Autodesk Fusion 360 part; units mm, degrees
(part 2 of 2)
  constraint parallel L118 L151
  constraint coincident P35 L167
  constraint coincident P35 L166
  constraint coincident P35 A26.centre
  constraint horizontal L165
  constraint perpendicular L135 L165
  constraint parallel L165 L187
  constraint parallel L128 L135
  constraint coincident P47 L131
  constraint coincident P47 L144
  constraint coincident P47 A24.centre
  constraint horizontal L111
  constraint perpendicular L108 L111
  constraint parallel L111 L113
  constraint parallel L108 L110
  constraint coincident P52 L114
  constraint coincident P52 L112
  constraint coincident P52 A18.centre
  constraint horizontal L115
  constraint perpendicular L115 L122
  constraint parallel L115 L117
  constraint parallel L121 L122
  constraint coincident P50 L119
  constraint coincident P50 L120
  constraint coincident P50 A19.centre
  constraint horizontal L116
  constraint perpendicular L116 L137
  constraint parallel L116 L180
  constraint parallel L136 L137
  constraint coincident P28 L134
  constraint coincident P28 L130
  constraint coincident P28 A21.centre
  constraint horizontal L161
  constraint perpendicular L161 L181
  constraint parallel L161 L164
  constraint parallel L181 L206
  constraint coincident P40 L154
  constraint coincident P40 L155
  constraint coincident P40 A29.centre
  constraint horizontal L195
  constraint perpendicular L195 L204
  constraint parallel L190 L195
  constraint parallel L194 L204
  constraint coincident P46 L197
  constraint coincident P46 L201
  constraint coincident P46 A34.centre
  constraint horizontal L193
  constraint perpendicular L186 L193
  constraint parallel L172 L193
  constraint parallel L175 L186
  constraint coincident P53 L189
  constraint coincident P53 L192
  constraint coincident P53 A33.centre
  constraint horizontal L216
  constraint perpendicular L216 L217
  constraint parallel L216 L218
  constraint parallel L217 L219
  constraint coincident L220 P56
  constraint coincident L221 P56
  constraint coincident P56 A36.centre
  measures "d3" distance of L1.end L2.end
  measures "d4" distance of L0.end L1.end
  measures "d5" diameter of A0
  measures "d6" distance of L6.end L7.end
  measures "d7" distance of L6.end L6.start
  measures "d8" diameter of A1
  measures "d9" distance of L14.end L12.end
  measures "d10" distance of L12.start L14.end
  measures "d11" diameter of A2
  measures "d12" distance of L31.start L28.end
  measures "d13" distance of L31.start L28.start
  measures "d14" diameter of A5
  measures "d15" distance of L24.end L20.start
  measures "d16" distance of L26.start L24.end
  measures "d17" diameter of A4
  measures "d18" distance of L18.start L18.end
  measures "d19" distance of L18.start L19.start
  measures "d20" diameter of A3
  measures "d21" distance of L50.end L65.start
  measures "d22" distance of L50.end L50.start
  measures "d23" diameter of A10
  measures "d24" distance of L57.end L59.end
  measures "d25" distance of L59.start L57.end
  measures "d26" diameter of A8
  measures "d27" distance of L37.end L38.end
  measures "d28" distance of L37.end L38.start
  measures "d29" diameter of A6
  measures "d30" distance of L46.start L46.end
  measures "d31" distance of L47.start L46.start
  measures "d32" diameter of A7
  measures "d33" distance of L45.start L45.end
  measures "d34" distance of L45.start L51.end
  measures "d35" diameter of A9
  measures "d36" distance of L36.end L42.end
  measures "d37" distance of L36.end L41.start
  measures "d38" diameter of A11
  measures "d39" distance of L76.start L74.end
  measures "d40" distance of L74.end L77.start
  measures "d41" diameter of A13
  measures "d42" distance of L73.start L73.end
  measures "d43" distance of L73.start L72.end
  measures "d44" diameter of A12
  measures "d45" distance of L78.start L84.end
  measures "d46" distance of L79.start L84.end
  measures "d47" diameter of A14
  measures "d48" distance of L91.end L97.end
  measures "d49" distance of L91.end L96.end
  measures "d50" diameter of A15
  measures "d51" distance of L98.end L98.start
  measures "d52" distance of L101.start L98.start
  measures "d53" diameter of A17
  measures "d54" distance of L94.end L92.end
  measures "d55" distance of L94.end L90.end
  measures "d56" diameter of A16
  measures "d57" distance of L183.end L185.end
  measures "d58" distance of L183.end L185.start
  measures "d59" diameter of A32
  measures "d60" distance of L200.end L203.end
  measures "d61" distance of L199.end L200.end
  measures "d62" diameter of A35
  measures "d63" distance of L139.end L132.end
  measures "d64" distance of L139.end L132.start
  measures "d65" diameter of A23
  measures "d66" distance of L170.start L170.end
  measures "d67" distance of L171.end L170.start
  measures "d68" diameter of A31
  measures "d69" distance of L205.start L205.end
  measures "d70" distance of L205.start L173.end
  measures "d71" diameter of A30
  measures "d72" distance of L125.end L140.start
  measures "d73" distance of L125.end L138.start
  measures "d74" diameter of A22
  measures "d75" distance of L124.start L147.start
  measures "d76" distance of L152.end L147.start
  measures "d77" diameter of A27
  measures "d78" distance of L145.end L145.start
  measures "d79" distance of L145.start L146.end
  measures "d80" diameter of A28
  measures "d81" distance of L126.end L127.start
  measures "d82" distance of L126.end L126.start
  measures "d83" diameter of A25
  measures "d84" distance of L109.start L123.end
  measures "d85" distance of L123.end L123.start
  measures "d86" diameter of A20
  measures "d87" distance of L151.end L118.start
  measures "d88" distance of L151.end L151.start
  measures "d89" diameter of A26
  measures "d90" distance of L128.start L131.end
  measures "d91" distance of L135.start L131.end
  measures "d92" diameter of A24
  measures "d93" distance of L108.end L110.start
  measures "d94" distance of L108.start L108.end
  measures "d95" diameter of A18
  measures "d96" distance of L117.start L117.end
  measures "d97" distance of L117.start L115.end
  measures "d98" diameter of A19
  measures "d99" distance of L134.end L130.end
  measures "d100" distance of L134.end L116.end
  measures "d101" diameter of A21
  measures "d102" distance of L155.end L154.end
  measures "d103" distance of L155.start L154.end
  measures "d104" diameter of A29
  measures "d105" distance of L190.end L190.start
  measures "d106" distance of L195.end L190.start
  measures "d107" diameter of A34
  measures "d108" distance of L172.end L172.start
  measures "d109" distance of L186.start L172.start
  measures "d110" diameter of A33
  measures "d111" distance of L217.end L218.end
  measures "d112" distance of L216.end L217.end
  measures "d113" diameter of A36
extrude "Extrude3" add sketch "basePCB" against normal blind 10.5 contours A0 makes body 1
extrude "Extrude4" add sketch "keys" along normal blind 3.8 contours L0 L1 L2 L3 | A0 | L6 L8 L9 L10 | A1 | L13 L15 L16 L17 | A2 | L18 L22 L23 L33 | A3 | L20 L25 L27 L30 | L29 L31 L32 L34 | A4 | A5 | A6 | L39 L40 L52 L54 | L41 L43 L44 L49 | L45 L51 L62 L63 | L46 L48 L53 L55 | A7 | A8 | L50 L65 L66 L70 | A9 | A10 | L60 L61 L64 L67 | A11 | L72 L73 L75 L87 | L76 L77 L80 L88 | A12 | A13 | L78 L82 L85 L86 | A14 | L90 L93 L95 L99 | A15 | A16 | L96 L97 L104 L107 | L98 L101 L102 L105 | A17 | L108 L110 L111 L113 | L109 L123 L160 L168 | A18 | L115 L117 L121 L122 | L116 L136 L137 L180 | L118 L151 L157 L163 | A19 | L124 L147 L152 L177 | A20 | L126 L127 L158 L159 | L128 L135 L165 L187 | A21 | A22 | L133 L141 L178 L202 | L138 L140 L176 L207 | A23 | A24 | A25 | A26 | L145 L146 L150 L212 | A27 | A28 | L161 L164 L181 L206 | A29 | L170 L171 L174 L179 | L172 L175 L186 L193 | L173 L205 L210 L214 | A30 | A31 | L188 L191 L196 L198 | L190 L194 L195 L204 | A32 | A33 | L199 L203 L209 L213 | A34 | A35 | L216 L217 L218 L219 | A36 bodies 1 makes body 2 at (-44.6574, 0, -22.3613) makes body 3 at (-36.7574, 0, -22.3613) makes body 4 at (-44.6574, 0, -9.9613) makes body 5 at (29.0426, 0, 5.6053) makes body 6 at (-10.6074, 0, -19.1947) makes body 7 at (29.0426, 0, -19.1947) makes body 8 at (21.1426, 0, 5.6053) makes body 9 at (10.7426, 0, -22.3613) makes body 10 at (18.6426, 0, 17.9053) makes body 11 at (13.2426, 0, -6.7947) makes body 12 at (13.2426, 0, 5.6053) makes body 13 at (-10.6074, 0, 17.9053) makes body 14 at (44.7926, 0, 5.6053) makes body 15 at (-10.6074, 0, -6.7947) makes body 16 at (-26.3574, 0, -6.7947) makes body 17 at (1.6397, 0, 27.6219) makes body 18 at (-34.2574, 0, -6.7947) makes body 19 at (-18.4574, 0, 17.9053) makes body 20 at (-18.4574, 0, 5.6053) makes body 21 at (-26.3574, 0, 5.6053) makes body 22 at (-42.1574, 0, 5.6053) makes body 23 at (44.7926, 0, -6.7947) makes body 24 at (-10.6074, 0, 5.6053) makes body 25 at (36.9426, 0, -19.1947) makes body 26 at (13.2426, 0, 17.9053) makes body 27 at (26.4926, 0, 17.9053) makes body 28 at (29.0426, 0, -6.7947) makes body 29 at (21.1426, 0, -6.7947) makes body 30 at (36.9426, 0, -6.7947) makes body 31 at (36.9426, 0, 5.6053) makes body 32 at (21.1426, 0, -19.1947) makes body 33 at (-28.8574, 0, -22.3613) makes body 34 at (-26.3574, 0, 17.9053) makes body 35 at (44.7926, 0, -19.1947) makes body 36 at (-34.2574, 0, 5.6053) makes body 37 at (-18.4574, 0, -19.1947) makes body 38 at (-18.4574, 0, -6.7947)
extrude "Extrude5" add sketch "keys" along normal blind 7.25 contours A0 | A1 | A2 | A3 | A4 | A5 | A6 | A7 | A8 | A9 | A10 | A11 | A12 | A13 | A14 | A15 | A16 | A17 | A18 | A19 | A20 | A21 | A22 | A23 | A24 | A25 | A26 | A27 | A28 | A29 | A30 | A31 | A32 | A33 | A34 | A35 | A36 bodies 2 3 4 5 6 7 8 9 10 11 12 13 14 15 16 17 18 19 20 21 22 23 24 25 26 27 28 29 30 31 32 33 34 35 36 37 38 1
sketch "base_v2pcb" plane through (0, 0, 0) normal (0, 1, 0) x (1, 0, 0)
  line L0 (39.648, 25.534) -> (39.898, 25.534)
  line L1 (39.898, 25.534) -> (46.898, 25.534)
  line L2 (47.148, 25.284) -> (47.148, 25.534)
  line L3 (39.648, 16.284) -> (39.648, 25.284)
  line L4 (47.148, 16.034) -> (47.148, 16.284)
  line L5 (46.898, 16.034) -> (39.898, 16.034)
  line L6 (47.148, 25.284) -> (47.148, 16.284)
  line L7 (39.898, 16.034) -> (39.648, 16.034)
  line L8 (39.648, 25.284) -> (39.648, 25.534)
  line L9 (39.648, 16.034) -> (39.648, 16.284)
  line L10 (47.148, 25.534) -> (46.898, 25.534)
  line L11 (31.774, -8.754) -> (31.774, -8.504)
  line L12 (32.024, -8.754) -> (31.774, -8.754)
  line L13 (31.774, 0.746) -> (32.024, 0.746)
  line L14 (39.274, -8.754) -> (39.274, -8.504)
  line L15 (46.898, 16.034) -> (47.148, 16.034)
  line L16 (39.274, 0.496) -> (39.274, -8.504)
  line L17 (31.774, -8.504) -> (31.774, 0.496)
  line L18 (32.024, 0.746) -> (39.024, 0.746)
  line L19 (31.774, 0.496) -> (31.774, 0.746)
  line L20 (-8.224, 16.034) -> (-8.224, 16.284)
  line L21 (-8.224, 0.746) -> (-8.474, 0.746)
  line L22 (-15.474, 0.746) -> (-8.474, 0.746)
  circle A0 centre (48.514, 33.79) radius 2.45
  circle A1 centre (-48.768, 33.79) radius 2.45
  line L23 (22.472, 35.136) -> (22.472, 31.936)
  line L24 (19.846, 28.48) -> (19.846, 31.48)
  circle A2 centre (-33.782, -33.52) radius 2.45
  circle A3 centre (-42.164, 31.492) radius 2.25
  line L25 (44.066, 33.002) -> (44.066, 36.102)
  line L26 (-23.402, 31.226) -> (-23.402, 28.226)
  line L27 (32.392, 35.136) -> (22.472, 35.136)
  line L28 (-11.142, 28.226) -> (-11.142, 31.226)
  line L29 (19.846, 32.036) -> (19.846, 35.036)
  line L30 (34.764, 28.226) -> (47.024, 28.226)
  line L31 (22.472, 31.936) -> (32.392, 31.936)
  line L32 (34.764, 31.226) -> (34.764, 28.226)
  line L33 (19.846, 35.036) -> (7.586, 35.036)
  line L34 (7.586, 32.036) -> (19.846, 32.036)
  line L35 (22.472, 28.38) -> (32.392, 28.38)
  line L36 (37.966, 36.102) -> (37.966, 33.002)
  line L37 (-11.142, 31.226) -> (-23.402, 31.226)
  line L38 (47.024, 28.226) -> (47.024, 31.226)
  line L39 (7.586, 35.036) -> (7.586, 32.036)
  line L40 (32.392, 31.58) -> (22.472, 31.58)
  line L41 (37.966, 33.002) -> (44.066, 33.002)
  line L42 (7.586, 31.48) -> (7.586, 28.48)
  line L43 (44.066, 36.102) -> (37.966, 36.102)
  line L44 (32.392, 31.936) -> (32.392, 35.136)
  circle A4 centre (33.782, -33.52) radius 2.45
  line L45 (32.392, 28.38) -> (32.392, 31.58)
  line L46 (7.586, 28.48) -> (19.846, 28.48)
  line L47 (47.024, 31.226) -> (34.764, 31.226)
  line L48 (19.846, 31.48) -> (7.586, 31.48)
  line L49 (22.472, 31.58) -> (22.472, 28.38)
  line L50 (-31.172, 35.268) -> (-31.172, 28.168)
  line L51 (-37.395, 28.295) -> (-34.995, 28.295)
  line L52 (-23.402, 28.226) -> (-11.142, 28.226)
  line L53 (-34.995, 28.295) -> (-34.995, 35.395)
  line L54 (-37.395, 35.395) -> (-37.395, 28.295)
  line L55 (-31.172, 28.168) -> (-28.772, 28.168)
  line L56 (-28.772, 35.268) -> (-31.172, 35.268)
  line L57 (-28.772, 28.168) -> (-28.772, 35.268)
  line L58 (-39.97, 3.588) -> (-46.97, 3.588)
  line L59 (-39.72, 3.588) -> (-39.72, 3.838)
  line L60 (-46.97, 13.088) -> (-39.97, 13.088)
  line L61 (-39.72, 12.838) -> (-39.72, 13.088)
  line L62 (-15.658, 35.34) -> (-15.658, 32.24)
  line L63 (-12.058, 32.24) -> (-12.058, 35.34)
  line L64 (-22.77, 32.24) -> (-19.17, 32.24)
  line L65 (-34.995, 35.395) -> (-37.395, 35.395)
  line L66 (-46.97, 3.588) -> (-47.22, 3.588)
  line L67 (-22.77, 35.34) -> (-22.77, 32.24)
  line L68 (-19.17, 35.34) -> (-22.77, 35.34)
  line L69 (-47.22, 13.088) -> (-46.97, 13.088)
  line L70 (-39.97, 3.588) -> (-39.72, 3.588)
  line L71 (-15.658, 32.24) -> (-12.058, 32.24)
  line L72 (-47.22, 3.838) -> (-47.22, 12.838)
  line L73 (-39.72, 13.088) -> (-39.97, 13.088)
  line L74 (-19.17, 32.24) -> (-19.17, 35.34)
  line L75 (-47.22, 3.588) -> (-47.22, 3.838)
  line L76 (-12.058, 35.34) -> (-15.658, 35.34)
  line L77 (-39.72, 12.838) -> (-39.72, 3.838)
  line L78 (39.274, 25.284) -> (39.274, 25.534)
  line L79 (31.774, 16.034) -> (31.774, 16.284)
  line L80 (32.024, 25.534) -> (39.024, 25.534)
  line L81 (31.774, 25.284) -> (31.774, 25.534)
  line L82 (39.024, 16.034) -> (39.274, 16.034)
  line L83 (32.024, 16.034) -> (31.774, 16.034)
  line L84 (31.774, 16.284) -> (31.774, 25.284)
  line L85 (31.774, 25.534) -> (32.024, 25.534)
  line L86 (31.4, 0.746) -> (31.15, 0.746)
  line L87 (39.274, 25.534) -> (39.024, 25.534)
  line L88 (24.15, -21.05) -> (23.9, -21.05)
  line L89 (23.9, -8.754) -> (23.9, -8.504)
  line L90 (31.4, -11.8) -> (31.4, -11.55)
  line L91 (31.4, -11.55) -> (31.15, -11.55)
  line L92 (24.15, -11.55) -> (31.15, -11.55)
  line L93 (39.274, 16.034) -> (39.274, 16.284)
  line L94 (23.9, -11.8) -> (23.9, -11.55)
  line L95 (23.9, 0.746) -> (24.15, 0.746)
  line L96 (23.9, -8.504) -> (23.9, 0.496)
  line L97 (23.9, -20.8) -> (23.9, -11.8)
  line L98 (31.4, 0.496) -> (31.4, -8.504)
  line L99 (23.9, -21.05) -> (23.9, -20.8)
  line L100 (31.4, -8.754) -> (31.4, -8.504)
  line L101 (31.4, -11.8) -> (31.4, -20.8)
  line L102 (24.15, 0.746) -> (31.15, 0.746)
  line L103 (31.15, -21.05) -> (31.4, -21.05)
  line L104 (39.024, 16.034) -> (32.024, 16.034)
  line L105 (23.9, -11.55) -> (24.15, -11.55)
  line L106 (23.9, 0.496) -> (23.9, 0.746)
  line L107 (24.15, -8.754) -> (23.9, -8.754)
  line L108 (31.4, 0.496) -> (31.4, 0.746)
  line L109 (31.15, -21.05) -> (24.15, -21.05)
  line L110 (31.4, -21.05) -> (31.4, -20.8)
  line L111 (31.15, -8.754) -> (31.4, -8.754)
  line L112 (31.472, 3.588) -> (31.472, 3.838)
  line L113 (23.972, 3.588) -> (23.972, 3.838)
  line L114 (24.222, 3.588) -> (23.972, 3.588)
  line L115 (31.222, 3.588) -> (24.222, 3.588)
  line L116 (31.15, -8.754) -> (24.15, -8.754)
  line L117 (24.222, 13.088) -> (31.222, 13.088)
  line L118 (23.972, 13.088) -> (24.222, 13.088)
  line L119 (23.972, 3.838) -> (23.972, 12.838)
  line L120 (31.472, 13.088) -> (31.222, 13.088)
  line L121 (31.222, 3.588) -> (31.472, 3.588)
  line L122 (23.972, 12.838) -> (23.972, 13.088)
  line L123 (31.472, 12.838) -> (31.472, 3.838)
  line L124 (31.472, 12.838) -> (31.472, 13.088)
  line L125 (23.9, 25.284) -> (23.9, 25.534)
  line L126 (31.4, 16.034) -> (31.4, 16.284)
  line L127 (31.15, 16.034) -> (24.15, 16.034)
  line L128 (24.15, 16.034) -> (23.9, 16.034)
  line L129 (16.026, -11.8) -> (16.026, -11.55)
  line L130 (23.9, 16.284) -> (23.9, 25.284)
  line L131 (31.4, 25.284) -> (31.4, 16.284)
  line L132 (31.4, 25.534) -> (31.15, 25.534)
  line L133 (16.026, -11.55) -> (16.276, -11.55)
  line L134 (24.15, 25.534) -> (31.15, 25.534)
  line L135 (31.4, 25.284) -> (31.4, 25.534)
  line L136 (23.9, 25.534) -> (24.15, 25.534)
  line L137 (23.9, 16.034) -> (23.9, 16.284)
  line L138 (31.15, 16.034) -> (31.4, 16.034)
  line L139 (-39.72, 16.034) -> (-39.72, 16.284)
  line L140 (23.526, -21.05) -> (23.526, -20.8)
  line L141 (23.526, 25.534) -> (23.276, 25.534)
  line L142 (-23.348, 0.746) -> (-16.348, 0.746)
  line L143 (-23.598, -11.8) -> (-23.598, -11.55)
  line L144 (-47.22, 25.284) -> (-47.22, 25.534)
  line L145 (23.526, -11.8) -> (23.526, -20.8)
  line L146 (23.526, 25.284) -> (23.526, 16.284)
  line L147 (23.276, 3.588) -> (23.526, 3.588)
  line L148 (23.526, 0.746) -> (23.276, 0.746)
  line L149 (-23.348, -11.55) -> (-16.348, -11.55)
  line L150 (16.026, 16.034) -> (16.026, 16.284)
  line L151 (-16.098, 0.496) -> (-16.098, -8.504)
  line L152 (23.526, -8.754) -> (23.526, -8.504)
  line L153 (23.526, -11.8) -> (23.526, -11.55)
  line L154 (23.526, 16.034) -> (23.526, 16.284)
  line L155 (-39.97, 16.034) -> (-39.72, 16.034)
  line L156 (23.276, -21.05) -> (16.276, -21.05)
  line L157 (16.026, 13.088) -> (16.276, 13.088)
  line L158 (16.026, 0.746) -> (16.276, 0.746)
  line L159 (16.026, 3.588) -> (16.026, 3.838)
  line L160 (16.026, -8.504) -> (16.026, 0.496)
  line L161 (23.526, 3.588) -> (23.526, 3.838)
  line L162 (-23.598, -21.05) -> (-23.598, -20.8)
  line L163 (16.276, -11.55) -> (23.276, -11.55)
  line L164 (-16.098, -11.55) -> (-16.348, -11.55)
  line L165 (16.276, 25.534) -> (23.276, 25.534)
  line L166 (-16.098, -11.8) -> (-16.098, -20.8)
  line L167 (-16.348, -21.05) -> (-16.098, -21.05)
  line L168 (23.526, 0.496) -> (23.526, -8.504)
  line L169 (-16.348, -8.754) -> (-16.098, -8.754)
  line L170 (23.526, 0.496) -> (23.526, 0.746)
  line L171 (-23.348, -21.05) -> (-23.598, -21.05)
  line L172 (-16.098, -11.8) -> (-16.098, -11.55)
  line L173 (16.026, -21.05) -> (16.026, -20.8)
  line L174 (16.026, 3.838) -> (16.026, 12.838)
  line L175 (23.526, -11.55) -> (23.276, -11.55)
  line L176 (-39.72, 25.284) -> (-39.72, 16.284)
  line L177 (-23.598, 0.746) -> (-23.348, 0.746)
  line L178 (23.276, -8.754) -> (16.276, -8.754)
  line L179 (-23.598, -8.754) -> (-23.598, -8.504)
  line L180 (-23.598, -11.55) -> (-23.348, -11.55)
  line L181 (16.276, 0.746) -> (23.276, 0.746)
  line L182 (16.276, 3.588) -> (16.026, 3.588)
  line L183 (23.526, 12.838) -> (23.526, 3.838)
  line L184 (16.026, 12.838) -> (16.026, 13.088)
  line L185 (-16.348, -8.754) -> (-23.348, -8.754)
  line L186 (23.276, -8.754) -> (23.526, -8.754)
  line L187 (-23.598, -8.504) -> (-23.598, 0.496)
  line L188 (23.276, 16.034) -> (16.276, 16.034)
  line L189 (16.026, -20.8) -> (16.026, -11.8)
  line L190 (16.276, -21.05) -> (16.026, -21.05)
  line L191 (-46.97, 25.534) -> (-39.97, 25.534)
  line L192 (-16.098, 0.746) -> (-16.348, 0.746)
  line L193 (16.276, 13.088) -> (23.276, 13.088)
  line L194 (-23.348, -8.754) -> (-23.598, -8.754)
  line L195 (-46.97, 16.034) -> (-47.22, 16.034)
  line L196 (23.526, 12.838) -> (23.526, 13.088)
  line L197 (23.276, 3.588) -> (16.276, 3.588)
  line L198 (16.026, -8.754) -> (16.026, -8.504)
  line L199 (-47.22, 16.284) -> (-47.22, 25.284)
  line L200 (16.026, 0.496) -> (16.026, 0.746)
  line L201 (23.276, 16.034) -> (23.526, 16.034)
  line L202 (16.276, -8.754) -> (16.026, -8.754)
  line L203 (23.526, 13.088) -> (23.276, 13.088)
  line L204 (16.026, 16.284) -> (16.026, 25.284)
  line L205 (23.276, -21.05) -> (23.526, -21.05)
  line L206 (-39.72, 25.534) -> (-39.97, 25.534)
  line L207 (-47.22, 16.034) -> (-47.22, 16.284)
  line L208 (-23.598, -20.8) -> (-23.598, -11.8)
  line L209 (23.526, 25.284) -> (23.526, 25.534)
  line L210 (-16.098, -21.05) -> (-16.098, -20.8)
  line L211 (-16.348, -21.05) -> (-23.348, -21.05)
  line L212 (16.026, 25.534) -> (16.276, 25.534)
  line L213 (16.276, 16.034) -> (16.026, 16.034)
  line L214 (-39.72, 25.284) -> (-39.72, 25.534)
  line L215 (-39.97, 16.034) -> (-46.97, 16.034)
  line L216 (16.026, 25.284) -> (16.026, 25.534)
  line L217 (-47.22, 25.534) -> (-46.97, 25.534)
  line L218 (-16.098, -8.754) -> (-16.098, -8.504)
  line L219 (-16.098, 0.496) -> (-16.098, 0.746)
  line L220 (-16.098, 13.088) -> (-16.348, 13.088)
  line L221 (-23.598, 0.496) -> (-23.598, 0.746)
  line L222 (-16.098, 12.838) -> (-16.098, 3.838)
  line L223 (-23.348, 13.088) -> (-16.348, 13.088)
  line L224 (-16.348, 3.588) -> (-23.348, 3.588)
  line L225 (-16.348, 3.588) -> (-16.098, 3.588)
  line L226 (-23.598, 3.838) -> (-23.598, 12.838)
  line L227 (-16.098, 3.588) -> (-16.098, 3.838)
  line L228 (-23.598, 3.588) -> (-23.598, 3.838)
  line L229 (-23.598, 13.088) -> (-23.348, 13.088)
  line L230 (-24.222, -21.05) -> (-23.972, -21.05)
  line L231 (-23.972, -11.8) -> (-23.972, -11.55)
  line L232 (-24.222, 3.588) -> (-23.972, 3.588)
  line L233 (-31.846, 12.838) -> (-31.846, 13.088)
  line L234 (-24.222, 16.034) -> (-23.972, 16.034)
  line L235 (-31.846, 25.284) -> (-31.846, 25.534)
  line L236 (-24.222, 16.034) -> (-31.222, 16.034)
  line L237 (-39.346, 16.034) -> (-39.346, 16.284)
  line L238 (-47.22, 12.838) -> (-47.22, 13.088)
  line L239 (-39.97, -8.754) -> (-46.97, -8.754)
  line L240 (-39.97, -8.754) -> (-39.72, -8.754)
  line L241 (-16.348, 16.034) -> (-16.098, 16.034)
  line L242 (-39.72, 0.496) -> (-39.72, -8.504)
  line L243 (-39.346, 0.496) -> (-39.346, 0.746)
  line L244 (-23.348, 25.534) -> (-16.348, 25.534)
  line L245 (-32.096, 16.034) -> (-31.846, 16.034)
  line L246 (-39.72, -8.754) -> (-39.72, -8.504)
  line L247 (-31.472, -20.8) -> (-31.472, -11.8)
  line L248 (-31.222, -8.754) -> (-31.472, -8.754)
  line L249 (-39.096, 3.588) -> (-39.346, 3.588)
  line L250 (-39.346, 16.284) -> (-39.346, 25.284)
  line L251 (-23.972, -8.754) -> (-23.972, -8.504)
  line L252 (-39.346, -8.754) -> (-39.346, -8.504)
  line L253 (-31.472, -11.55) -> (-31.222, -11.55)
  line L254 (-31.222, 13.088) -> (-24.222, 13.088)
  line L255 (-32.096, 16.034) -> (-39.096, 16.034)
  line L256 (-31.846, 16.034) -> (-31.846, 16.284)
  line L257 (-31.222, 3.588) -> (-31.472, 3.588)
  line L258 (-31.846, 12.838) -> (-31.846, 3.838)
  line L259 (-31.472, 3.588) -> (-31.472, 3.838)
  line L260 (-16.098, 25.534) -> (-16.348, 25.534)
  line L261 (-31.472, 0.496) -> (-31.472, 0.746)
  line L262 (-16.348, 16.034) -> (-23.348, 16.034)
  line L263 (-31.846, 13.088) -> (-32.096, 13.088)
  line L264 (-23.598, 16.284) -> (-23.598, 25.284)
  line L265 (-39.346, 12.838) -> (-39.346, 13.088)
  line L266 (-47.22, -8.754) -> (-47.22, -8.504)
  line L267 (-16.098, 25.284) -> (-16.098, 16.284)
  line L268 (-39.72, 0.746) -> (-39.97, 0.746)
  line L269 (-31.222, 25.534) -> (-24.222, 25.534)
  line L270 (-23.972, 0.496) -> (-23.972, -8.504)
  line L271 (-31.472, 25.534) -> (-31.222, 25.534)
  line L272 (-39.346, -8.504) -> (-39.346, 0.496)
  line L273 (-23.972, 12.838) -> (-23.972, 13.088)
  line L274 (-39.096, 13.088) -> (-32.096, 13.088)
  line L275 (-39.096, 16.034) -> (-39.346, 16.034)
  line L276 (-47.22, -8.504) -> (-47.22, 0.496)
  line L277 (-24.222, -8.754) -> (-31.222, -8.754)
  line L278 (-31.846, 3.588) -> (-31.846, 3.838)
  line L279 (-31.846, 0.746) -> (-32.096, 0.746)
  line L280 (-31.846, 0.496) -> (-31.846, 0.746)
  line L281 (-23.972, 12.838) -> (-23.972, 3.838)
  line L282 (-32.096, -8.754) -> (-31.846, -8.754)
  line L283 (-23.598, 25.284) -> (-23.598, 25.534)
  line L284 (-32.096, 3.588) -> (-39.096, 3.588)
  line L285 (-31.472, 0.746) -> (-31.222, 0.746)
  line L286 (-23.972, 0.746) -> (-24.222, 0.746)
  line L287 (-31.472, 12.838) -> (-31.472, 13.088)
  line L288 (-23.598, 16.034) -> (-23.598, 16.284)
  line L289 (-24.222, 3.588) -> (-31.222, 3.588)
  line L290 (-31.472, 16.284) -> (-31.472, 25.284)
  line L291 (-23.598, 12.838) -> (-23.598, 13.088)
  line L292 (-23.972, 3.588) -> (-23.972, 3.838)
  line L293 (-23.972, 25.284) -> (-23.972, 16.284)
  line L294 (-39.346, 25.284) -> (-39.346, 25.534)
  line L295 (-31.222, 0.746) -> (-24.222, 0.746)
  line L296 (-23.972, -11.55) -> (-24.222, -11.55)
  line L297 (-16.098, 12.838) -> (-16.098, 13.088)
  line L298 (-31.472, -8.504) -> (-31.472, 0.496)
  line L299 (-39.346, 25.534) -> (-39.096, 25.534)
  line L300 (-31.472, -11.8) -> (-31.472, -11.55)
  line L301 (-31.846, 0.496) -> (-31.846, -8.504)
  line L302 (-39.096, -8.754) -> (-39.346, -8.754)
  line L303 (-23.972, 16.034) -> (-23.972, 16.284)
  line L304 (-23.348, 16.034) -> (-23.598, 16.034)
  line L305 (-32.096, 3.588) -> (-31.846, 3.588)
  line L306 (-23.598, 25.534) -> (-23.348, 25.534)
  line L307 (-39.346, 3.838) -> (-39.346, 12.838)
  line L308 (-23.348, 3.588) -> (-23.598, 3.588)
  line L309 (-31.472, 13.088) -> (-31.222, 13.088)
  line L310 (-31.472, 3.838) -> (-31.472, 12.838)
  line L311 (-31.846, -8.754) -> (-31.846, -8.504)
  line L312 (-16.098, 25.284) -> (-16.098, 25.534)
  line L313 (-23.972, -11.8) -> (-23.972, -20.8)
  line L314 (-23.972, 25.284) -> (-23.972, 25.534)
  line L315 (-31.222, -11.55) -> (-24.222, -11.55)
  line L316 (-39.096, 0.746) -> (-32.096, 0.746)
  line L317 (-23.972, 0.496) -> (-23.972, 0.746)
  line L318 (-31.472, 25.284) -> (-31.472, 25.534)
  line L319 (-39.346, 3.588) -> (-39.346, 3.838)
  line L320 (-47.22, 0.496) -> (-47.22, 0.746)
  line L321 (-39.096, 25.534) -> (-32.096, 25.534)
  line L322 (-39.346, 0.746) -> (-39.096, 0.746)
  line L323 (-31.472, -21.05) -> (-31.472, -20.8)
  line L324 (-32.096, -8.754) -> (-39.096, -8.754)
  line L325 (-31.472, 16.034) -> (-31.472, 16.284)
  line L326 (-31.846, 25.534) -> (-32.096, 25.534)
  line L327 (-23.972, -21.05) -> (-23.972, -20.8)
  line L328 (-31.222, 16.034) -> (-31.472, 16.034)
  line L329 (-23.972, 13.088) -> (-24.222, 13.088)
  line L330 (-47.22, 0.746) -> (-46.97, 0.746)
  line L331 (-46.97, -8.754) -> (-47.22, -8.754)
  line L332 (-16.098, 16.034) -> (-16.098, 16.284)
  line L333 (-39.346, 13.088) -> (-39.096, 13.088)
  line L334 (-24.222, -8.754) -> (-23.972, -8.754)
  line L335 (-46.97, 0.746) -> (-39.97, 0.746)
  line L336 (-24.222, -21.05) -> (-31.222, -21.05)
  line L337 (-39.72, 0.496) -> (-39.72, 0.746)
  line L338 (-23.972, 25.534) -> (-24.222, 25.534)
  line L339 (-31.472, -8.754) -> (-31.472, -8.504)
  line L340 (-31.222, -21.05) -> (-31.472, -21.05)
  line L341 (-31.846, 25.284) -> (-31.846, 16.284)
  line L342 (-15.474, -21.05) -> (-15.724, -21.05)
  line L343 (-15.724, 16.284) -> (-15.724, 25.284)
  line L344 (8.152, 3.588) -> (8.152, 3.838)
  line L345 (-8.224, 25.284) -> (-8.224, 25.534)
  line L346 (-15.724, 25.534) -> (-15.474, 25.534)
  line L347 (15.652, 12.838) -> (15.652, 3.838)
  line L348 (15.402, 3.588) -> (8.402, 3.588)
  line L349 (8.402, 25.534) -> (15.402, 25.534)
  line L350 (-8.474, -21.05) -> (-8.224, -21.05)
  line L351 (-15.474, 3.588) -> (-15.724, 3.588)
  line L352 (-15.724, -20.8) -> (-15.724, -11.8)
  line L353 (-8.474, -21.05) -> (-15.474, -21.05)
  line L354 (-8.474, 3.588) -> (-15.474, 3.588)
  line L355 (8.152, 3.838) -> (8.152, 12.838)
  line L356 (-8.474, 16.034) -> (-8.224, 16.034)
  line L357 (15.652, 13.088) -> (15.402, 13.088)
  line L358 (-8.224, -11.55) -> (-8.474, -11.55)
  line L359 (-8.224, 25.284) -> (-8.224, 16.284)
  line L360 (8.152, 25.534) -> (8.402, 25.534)
  line L361 (8.402, 13.088) -> (15.402, 13.088)
  line L362 (-15.724, 3.838) -> (-15.724, 12.838)
  line L363 (-15.724, 16.034) -> (-15.724, 16.284)
  line L364 (-8.224, -21.05) -> (-8.224, -20.8)
  line L365 (-8.224, 25.534) -> (-8.474, 25.534)
  line L366 (-15.474, -11.55) -> (-8.474, -11.55)
  line L367 (15.402, 16.034) -> (8.402, 16.034)
  line L368 (15.652, 25.284) -> (15.652, 25.534)
  line L369 (-15.724, 13.088) -> (-15.474, 13.088)
  line L370 (8.402, 16.034) -> (8.152, 16.034)
  line L371 (-8.224, -11.8) -> (-8.224, -20.8)
  line L372 (15.402, 16.034) -> (15.652, 16.034)
  line L373 (15.402, 3.588) -> (15.652, 3.588)
  line L374 (-15.724, 25.284) -> (-15.724, 25.534)
  line L375 (-8.224, 12.838) -> (-8.224, 3.838)
  line L376 (-15.724, 3.588) -> (-15.724, 3.838)
  line L377 (15.652, 25.534) -> (15.402, 25.534)
  line L378 (8.152, 25.284) -> (8.152, 25.534)
  line L379 (-15.724, -21.05) -> (-15.724, -20.8)
  line L380 (8.152, 13.088) -> (8.402, 13.088)
  line L381 (-15.724, 12.838) -> (-15.724, 13.088)
  line L382 (-8.224, 12.838) -> (-8.224, 13.088)
  line L383 (-8.474, 16.034) -> (-15.474, 16.034)
  line L384 (-15.474, 13.088) -> (-8.474, 13.088)
  line L385 (-8.474, 3.588) -> (-8.224, 3.588)
  line L386 (8.152, 16.284) -> (8.152, 25.284)
  line L387 (-8.224, 3.588) -> (-8.224, 3.838)
  line L388 (-15.474, 16.034) -> (-15.724, 16.034)
  line L389 (-15.474, 25.534) -> (-8.474, 25.534)
  line L390 (-15.724, -11.8) -> (-15.724, -11.55)
  line L391 (8.152, 12.838) -> (8.152, 13.088)
  line L392 (-8.224, -11.8) -> (-8.224, -11.55)
  line L393 (8.152, 16.034) -> (8.152, 16.284)
  line L394 (15.652, 3.588) -> (15.652, 3.838)
  line L395 (-15.724, -11.55) -> (-15.474, -11.55)
  line L396 (15.652, 25.284) -> (15.652, 16.284)
  line L397 (15.652, 16.034) -> (15.652, 16.284)
  line L398 (-8.224, 13.088) -> (-8.474, 13.088)
  line L399 (8.402, 3.588) -> (8.152, 3.588)
  line L400 (15.652, 12.838) -> (15.652, 13.088)
  line L401 (8.152, -20.8) -> (8.152, -11.8)
  line L402 (8.402, 0.746) -> (15.402, 0.746)
  line L403 (39.648, 3.588) -> (39.648, 3.838)
  line L404 (8.402, -8.754) -> (8.152, -8.754)
  line L405 (15.402, -8.754) -> (8.402, -8.754)
  line L406 (15.652, -11.8) -> (15.652, -20.8)
  line L407 (39.648, 12.838) -> (39.648, 13.088)
  line L408 (39.898, 3.588) -> (39.648, 3.588)
  line L409 (15.652, 0.496) -> (15.652, -8.504)
  line L410 (39.648, 3.838) -> (39.648, 12.838)
  line L411 (47.148, 3.588) -> (47.148, 3.838)
  line L412 (8.152, -8.754) -> (8.152, -8.504)
  line L413 (15.652, 0.746) -> (15.402, 0.746)
  line L414 (15.652, -11.55) -> (15.402, -11.55)
  line L415 (47.148, 12.838) -> (47.148, 3.838)
  line L416 (8.402, -11.55) -> (15.402, -11.55)
  line L417 (46.898, -8.754) -> (39.898, -8.754)
  line L418 (46.898, 3.588) -> (39.898, 3.588)
  line L419 (8.152, -8.504) -> (8.152, 0.496)
  line L420 (15.402, -21.05) -> (15.652, -21.05)
  line L421 (47.148, 0.496) -> (47.148, 0.746)
  line L422 (8.152, -11.55) -> (8.402, -11.55)
  line L423 (4.89, -5.078) -> (4.89, 31.022)
  line L424 (-4.91, -5.078) -> (4.89, -5.078)
  line L425 (47.148, 0.746) -> (46.898, 0.746)
  line L426 (15.652, -8.754) -> (15.652, -8.504)
  line L427 (8.152, 0.746) -> (8.402, 0.746)
  line L428 (15.652, -21.05) -> (15.652, -20.8)
  line L429 (39.648, -8.754) -> (39.648, -8.504)
  line L430 (46.898, 3.588) -> (47.148, 3.588)
  line L431 (8.152, -11.8) -> (8.152, -11.55)
  line L432 (47.148, 13.088) -> (46.898, 13.088)
  line L433 (39.898, -8.754) -> (39.648, -8.754)
  line L434 (46.898, -8.754) -> (47.148, -8.754)
  line L435 (39.648, 0.496) -> (39.648, 0.746)
  line L436 (39.648, 0.746) -> (39.898, 0.746)
  line L437 (39.898, 0.746) -> (46.898, 0.746)
  line L438 (8.402, -21.05) -> (8.152, -21.05)
  line L439 (47.148, -8.754) -> (47.148, -8.504)
  line L440 (15.652, 0.496) -> (15.652, 0.746)
  line L441 (39.648, -8.504) -> (39.648, 0.496)
  line L442 (8.152, 0.496) -> (8.152, 0.746)
  line L443 (15.652, -11.8) -> (15.652, -11.55)
  line L444 (8.152, -21.05) -> (8.152, -20.8)
  line L445 (15.402, -21.05) -> (8.402, -21.05)
  line L446 (4.89, 31.022) -> (-4.91, 31.022)
  line L447 (47.148, 12.838) -> (47.148, 13.088)
  line L448 (39.648, 13.088) -> (39.898, 13.088)
  line L449 (39.898, 13.088) -> (46.898, 13.088)
  line L450 (47.148, 0.496) -> (47.148, -8.504)
  line L451 (-4.91, 31.022) -> (-4.91, -5.078)
  line L452 (15.402, -8.754) -> (15.652, -8.754)
  line L453 (-3.536, -12.15) -> (-3.536, -16.75)
  line L454 (-3.536, -16.75) -> (-1.036, -16.75)
  line L455 (-1.036, -16.75) -> (-1.036, -12.15)
  line L456 (-1.036, -12.15) -> (-3.536, -12.15)
  line L457 (-5.86, -6.082) -> (-5.86, -11.682)
  line L458 (6.04, -6.082) -> (-5.86, -6.082)
  line L459 (-5.86, -11.682) -> (6.04, -11.682)
  line L460 (3.79, -12.15) -> (1.29, -12.15)
  line L461 (3.79, -16.75) -> (3.79, -12.15)
  line L462 (6.04, -11.682) -> (6.04, -6.082)
  line L463 (1.29, -12.15) -> (1.29, -16.75)
  line L464 (1.29, -16.75) -> (3.79, -16.75)
  line L465 (-15.724, 0.746) -> (-15.474, 0.746)
  line L466 (-15.724, -8.504) -> (-15.724, 0.496)
  line L467 (-8.224, -8.754) -> (-8.224, -8.504)
  line L468 (-15.474, -8.754) -> (-15.724, -8.754)
  line L469 (-8.224, 0.496) -> (-8.224, -8.504)
  line L470 (-8.474, -8.754) -> (-8.224, -8.754)
  line L471 (-15.724, -8.754) -> (-15.724, -8.504)
  line L472 (-8.474, -8.754) -> (-15.474, -8.754)
  line L473 (-8.224, 0.496) -> (-8.224, 0.746)
  line L474 (-15.724, 0.496) -> (-15.724, 0.746)
  line L475 (39.346, 12.838) -> (39.346, 13.088)
  line L476 (39.024, -8.754) -> (39.274, -8.754)
  line L477 (39.024, -8.754) -> (32.024, -8.754)
  line L478 (39.274, 0.496) -> (39.274, 0.746)
  line L479 (39.274, 0.746) -> (39.024, 0.746)
  line L480 (39.346, 3.588) -> (39.346, 3.838)
  line L481 (31.846, 3.588) -> (31.846, 3.838)
  line L482 (32.096, 3.588) -> (31.846, 3.588)
  line L483 (39.346, 12.838) -> (39.346, 3.838)
  line L484 (39.346, 13.088) -> (39.096, 13.088)
  line L485 (32.096, 13.088) -> (39.096, 13.088)
  line L486 (31.846, 13.088) -> (32.096, 13.088)
  line L487 (39.096, 3.588) -> (32.096, 3.588)
  line L488 (39.096, 3.588) -> (39.346, 3.588)
  line L489 (31.846, 3.838) -> (31.846, 12.838)
  line L490 (31.846, 12.838) -> (31.846, 13.088)
  line L491 (39.274, 25.284) -> (39.274, 16.284)
  arc A5 (35.306, -37.584) -> (36.068, -37.33) centre (35.306, -36.314) ccw
  arc A6 (-51.308, 37.6) -> (-52.578, 36.33) centre (-51.308, 36.33) ccw
  line L492 (52.07, -21.328) -> (36.068, -37.33)
  line L493 (-52.578, -20.566) -> (-52.578, 36.33)
  arc A7 (52.07, -21.328) -> (52.324, -20.566) centre (51.054, -20.566) ccw
  arc A8 (-36.322, -37.33) -> (-35.56, -37.584) centre (-35.56, -36.314) ccw
  line L494 (-51.308, 37.6) -> (51.054, 37.6)
  arc A9 (-52.578, -20.566) -> (-52.324, -21.328) centre (-51.308, -20.566) ccw
  line L495 (-36.322, -37.33) -> (-52.324, -21.328)
  line L496 (52.324, 36.33) -> (52.324, -20.566)
  line L497 (35.306, -37.584) -> (-35.56, -37.584)
  arc A10 (52.324, 36.33) -> (51.054, 37.6) centre (51.054, 36.33) ccw
  circle A11 centre (-33.782, -33.52) radius 1.25
  circle A12 centre (33.782, -33.52) radius 1.25
  circle A13 centre (-48.668, 33.784) radius 1.25
  circle A14 centre (48.614, 33.784) radius 1.25
  dimension "d128" = 2.5
  dimension "d129" = 2.5
  constraint concentric A2 A11
  constraint concentric A4 A12
  measures "d128" diameter of A11
  measures "d129" diameter of A12
extrude "Extrude6" add sketch "base_v2pcb" against normal blind 1.6 contours L0 L1 L2 L3 L4 L5 L6 L7 L8 L9 L10 L15 | L11 L12 L13 L14 L16 L17 L18 L19 L476 L477 L478 L479 | L20 L343 L345 L346 L356 L359 L363 L365 L374 L383 L388 L389 | L21 L22 L465 L466 L467 L468 L469 L470 L471 L472 L473 L474 | A0 | A1 | L23 L27 L31 L44 | L24 L42 L46 L48 | A2 | A3 | L25 L36 L41 L43 | L26 L28 L37 L52 | L29 L33 L34 L39 | L30 L32 L38 L47 | L35 L40 L45 L49 | A4 | L50 L55 L56 L57 | L51 L53 L54 L65 | L58 L59 L60 L61 L66 L69 L70 L72 L73 L75 L77 L238 | L62 L63 L71 L76 | L64 L67 L68 L74 | L78 L79 L80 L81 L82 L83 L84 L85 L87 L93 L104 L491 | L86 L89 L95 L96 L98 L100 L102 L106 L107 L108 L111 L116 | L88 L90 L91 L92 L94 L97 L99 L101 L103 L105 L109 L110 | L112 L113 L114 L115 L117 L118 L119 L120 L121 L122 L123 L124 | L125 L126 L127 L128 L130 L131 L132 L134 L135 L136 L137 L138 | L129 L133 L140 L145 L153 L156 L163 L173 L175 L189 L190 L205 | L139 L144 L155 L176 L191 L195 L199 L206 L207 L214 L215 L217 | L141 L146 L150 L154 L165 L188 L201 L204 L209 L212 L213 L216 | L142 L151 L169 L177 L179 L185 L187 L192 L194 L218 L219 L221 | L143 L149 L162 L164 L166 L167 L171 L172 L180 L208 L210 L211 | L147 L157 L159 L161 L174 L182 L183 L184 L193 L196 L197 L203 | L148 L152 L158 L160 L168 L170 L178 L181 L186 L198 L200 L202 | L220 L222 L223 L224 L225 L226 L227 L228 L229 L291 L297 L308 | L230 L231 L247 L253 L296 L300 L313 L315 L323 L327 L336 L340 | L232 L254 L257 L259 L273 L281 L287 L289 L292 L309 L310 L329 | L233 L249 L258 L263 L265 L274 L278 L284 L305 L307 L319 L333 | L234 L236 L269 L271 L290 L293 L303 L314 L318 L325 L328 L338 | L235 L237 L245 L250 L255 L256 L275 L294 L299 L321 L326 L341 | L239 L240 L242 L246 L266 L268 L276 L320 L330 L331 L335 L337 | L241 L244 L260 L262 L264 L267 L283 L288 L304 L306 L312 L332 | L243 L252 L272 L279 L280 L282 L301 L302 L311 L316 L322 L324 | L248 L251 L261 L270 L277 L285 L286 L295 L298 L317 L334 L339 | L342 L350 L352 L353 L358 L364 L366 L371 L379 L390 L392 L395 | L344 L347 L348 L355 L357 L361 L373 L380 L391 L394 L399 L400 | L349 L360 L367 L368 L370 L372 L377 L378 L386 L393 L396 L397 | L351 L354 L362 L369 L375 L376 L381 L382 L384 L385 L387 L398 | L401 L406 L414 L416 L420 L422 L428 L431 L438 L443 L444 L445 | L402 L404 L405 L409 L412 L413 L419 L426 L427 L440 L442 L452 | L403 L407 L408 L410 L411 L415 L418 L430 L432 L447 L448 L449 | L417 L421 L425 L429 L433 L434 L435 L436 L437 L439 L441 L450 | L423 L424 L446 L451 | L453 L454 L455 L456 | L457 L458 L459 L462 | L460 L461 L463 L464 | L475 L480 L481 L482 L483 L484 L485 L486 L487 L488 L489 L490 | A5 A6 L492 L493 A7 A8 L494 A9 L495 L496 L497 A10 bodies 1 2 3 4 5 6 7 8 9 10 11 12 13 14 15 16 17 18 19 20 21 22 23 24 25 26 27 28 29 30 31 32 33 34 35 36 37 38
extrude "Extrude7" add sketch "base_v2pcb" along normal blind 1 from surface at 4 separate body contours L0 L1 L2 L3 L4 L5 L6 L7 L8 L9 L10 L15 | L11 L12 L13 L14 L16 L17 L18 L19 L476 L477 L478 L479 | L20 L343 L345 L346 L356 L359 L363 L365 L374 L383 L388 L389 | L21 L22 L465 L466 L467 L468 L469 L470 L471 L472 L473 L474 | A0 | A1 | L23 L27 L31 L44 | L24 L42 L46 L48 | A2 | A3 | L25 L36 L41 L43 | L26 L28 L37 L52 | L29 L33 L34 L39 | L30 L32 L38 L47 | L35 L40 L45 L49 | A4 | L50 L55 L56 L57 | L51 L53 L54 L65 | L58 L59 L60 L61 L66 L69 L70 L72 L73 L75 L77 L238 | L62 L63 L71 L76 | L64 L67 L68 L74 | L78 L79 L80 L81 L82 L83 L84 L85 L87 L93 L104 L491 | L86 L89 L95 L96 L98 L100 L102 L106 L107 L108 L111 L116 | L88 L90 L91 L92 L94 L97 L99 L101 L103 L105 L109 L110 | L112 L113 L114 L115 L117 L118 L119 L120 L121 L122 L123 L124 | L125 L126 L127 L128 L130 L131 L132 L134 L135 L136 L137 L138 | L129 L133 L140 L145 L153 L156 L163 L173 L175 L189 L190 L205 | L139 L144 L155 L176 L191 L195 L199 L206 L207 L214 L215 L217 | L141 L146 L150 L154 L165 L188 L201 L204 L209 L212 L213 L216 | L142 L151 L169 L177 L179 L185 L187 L192 L194 L218 L219 L221 | L143 L149 L162 L164 L166 L167 L171 L172 L180 L208 L210 L211 | L147 L157 L159 L161 L174 L182 L183 L184 L193 L196 L197 L203 | L148 L152 L158 L160 L168 L170 L178 L181 L186 L198 L200 L202 | L220 L222 L223 L224 L225 L226 L227 L228 L229 L291 L297 L308 | L230 L231 L247 L253 L296 L300 L313 L315 L323 L327 L336 L340 | L232 L254 L257 L259 L273 L281 L287 L289 L292 L309 L310 L329 | L233 L249 L258 L263 L265 L274 L278 L284 L305 L307 L319 L333 | L234 L236 L269 L271 L290 L293 L303 L314 L318 L325 L328 L338 | L235 L237 L245 L250 L255 L256 L275 L294 L299 L321 L326 L341 | L239 L240 L242 L246 L266 L268 L276 L320 L330 L331 L335 L337 | L241 L244 L260 L262 L264 L267 L283 L288 L304 L306 L312 L332 | L243 L252 L272 L279 L280 L282 L301 L302 L311 L316 L322 L324 | L248 L251 L261 L270 L277 L285 L286 L295 L298 L317 L334 L339 | L342 L350 L352 L353 L358 L364 L366 L371 L379 L390 L392 L395 | L344 L347 L348 L355 L357 L361 L373 L380 L391 L394 L399 L400 | L349 L360 L367 L368 L370 L372 L377 L378 L386 L393 L396 L397 | L351 L354 L362 L369 L375 L376 L381 L382 L384 L385 L387 L398 | L401 L406 L414 L416 L420 L422 L428 L431 L438 L443 L444 L445 | L402 L404 L405 L409 L412 L413 L419 L426 L427 L440 L442 L452 | L403 L407 L408 L410 L411 L415 L418 L430 L432 L447 L448 L449 | L417 L421 L425 L429 L433 L434 L435 L436 L437 L439 L441 L450 | L453 L454 L455 L456 | L457 L458 L459 L462 | L460 L461 L463 L464 | L475 L480 L481 L482 L483 L484 L485 L486 L487 L488 L489 L490 | A5 A6 L492 L493 A7 A8 L494 A9 L495 L496 L497 A10 makes body 39
named bodies: "keyboard_pcb", "cover_pcb"
